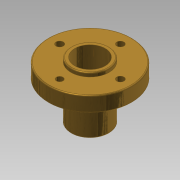
# Autodesk Inventor part: Z Akse gevindstang møtrik
Saved by Autodesk Inventor 2016 (Build 200138000, 138)
## iProperties
Created: 2015-06-04
Part Number: Z Akse gevindstang møtrik
Material: Brass, Soft Yellow
Document SubType Name: Modeling
Designer: Mathias L. Kjeldgaard
Density: 8.47 g/cm^3
Appearance: Brass - Satin
Mass: 13.4216 g
Surface Area: 17.086 cm^2
Volume: 1.58461 cm^3
Author: Mathias L. Kjeldgaard
Autodesk Inventor part; units mm, degrees
ref_plane "YZ Plane" through (0, 0, 0) normal (1, 0, 0) x (0, 1, 0)
ref_plane "XZ Plane" through (0, 0, 0) normal (0, 1, 0) x (-1, 0, 0)
ref_plane "XY Plane" through (0, 0, 0) normal (0, 0, 1) x (1, 0, 0)
sketch "Sketch1" plane through (0, 0, 0) normal (0, 0, 1) x (1, 0, 0)
  circle A0 centre (0, 0) radius 11
  circle A1 centre (0, 0) radius 4
  dimension "d0" = 22
  dimension "d3" = 8
  constraints: 2 centre point, 2 coincident
  measures "d0" diameter of A0
  measures "d3" diameter of A1
extrude "Extrusion2" add sketch "Sketch1" along normal mid plane 4
sketch "Sketch2" plane through (0, 0, 2) normal (0, 0, 1) x (1, 0, 0)
  circle A0 centre (0, 0) radius 4 projected
  circle A1 centre (0, 0) radius 11 projected
  circle A2 centre (0, 0) radius 5
  circle A3 centre (0, 0) radius 4
  dimension "d6" = 10
  dimension "d7" = 8
  constraints: 2 centre point, 2 coincident
  measures "d6" diameter of A2
  measures "d7" diameter of A3
extrude "Extrusion3" add sketch "Sketch2" along normal blind 1 contours A2
sketch "Sketch3" plane through (0, 0, 2) normal (0, 0, 1) x (1, 0, 0)
  circle A0 centre (0, 0) radius 5 projected
  circle A1 centre (0, -8) radius 0.8657
  circle A2 centre (8, 0) radius 0.9464
  circle A3 centre (0, 8) radius 0.9341
  circle A4 centre (-8, 0) radius 0.9592
  dimension "d10" = 8
  dimension "d11" = 8
  dimension "d12" = 8
  dimension "d13" = 8
  constraints: 4 centre point
  measures "d10" distance of A0.centre A4.centre
  measures "d11" distance of A2.centre A0.centre
  measures "d12" distance of A0.centre A3.centre
  measures "d13" distance of A0.centre A1.centre
extrude "Extrusion4" cut sketch "Sketch3" against normal up to surface (4 mm away) contours A1 | A2 | A3 | A4
sketch "Sketch4" plane through (0, 0, -2) normal (0, 0, -1) x (-1, 0, 0)
  circle A0 centre (0, 0) radius 4 projected
  circle A1 centre (0, 0) radius 11 projected
  circle A2 centre (0, 0) radius 4
  circle A3 centre (0, 0) radius 5
  dimension "d16" = 10
  constraints: 2 centre point, 2 coincident, 1 concentric
  measures "d16" diameter of A3
extrude "Extrusion5" add sketch "Sketch4" along normal blind 10 contours A3
fillet "Fillet1" radius 0.25 4 edges at (-11, 0, -2) (-11, 0, 2) (5, 0, -12) (-5, 0, 3)
body "Solid2"
